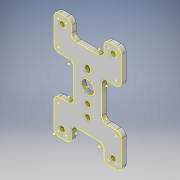
# Autodesk Inventor part: TapaInferior
Saved by Autodesk Inventor 2019 (Build 230136000, 136)
## iProperties
Created: 2019-03-04
Part Number: TapaInferior
Material: Generic
Document SubType Name: Modeling
Designer: Kenny
Density: 1 g/cm^3
Appearance: Default
Author: Kenny
Autodesk Inventor part; units mm, degrees
ref_plane "YZ Plane" through (0, 0, 0) normal (1, 0, 0) x (0, 1, 0)
ref_plane "XZ Plane" through (0, 0, 0) normal (0, 1, 0) x (-1, 0, 0)
ref_plane "XY Plane" through (0, 0, 0) normal (0, 0, 1) x (1, 0, 0)
sketch "Sketch1" plane through (0, 0, 0) normal (0, 0, 1) x (1, 0, 0)
  line L0 (41, 0) -> (41, 65.3) construction
  line L1 (0, 65.3) -> (0, 0) construction
  line L2 (41, 0) -> (41, 21)
  line L3 (0, 21) -> (0, 0)
  line L4 (41, 65.3) -> (41, 44.3)
  line L5 (0, 44.3) -> (0, 65.3)
  line L6 (29, 44.3) -> (29, 21)
  line L7 (12, 21) -> (12, 44.3)
  line L8 (41, 44.3) -> (29, 44.3)
  line L9 (12, 44.3) -> (0, 44.3)
  line L10 (41, 21) -> (29, 21)
  line L11 (12, 21) -> (0, 21)
  line L12 (30.5, 65.3) -> (30.5, 55.3)
  line L13 (30.5, 55.3) -> (10.5, 55.3)
  line L14 (10.5, 55.3) -> (10.5, 65.3)
  line L15 (41, 65.3) -> (30.5, 65.3) construction
  line L16 (10.5, 65.3) -> (0, 65.3) construction
  line L17 (0, 65.3) -> (10.5, 65.3)
  line L18 (30.5, 65.3) -> (41, 65.3)
  line L19 (10.5, 0) -> (10.5, 10)
  line L20 (10.5, 10) -> (30.5, 10)
  line L21 (30.5, 10) -> (30.5, 0)
  line L22 (0, 0) -> (10.5, 0) construction
  line L23 (30.5, 0) -> (41, 0) construction
  line L24 (0, 0) -> (10.5, 0)
  line L25 (30.5, 0) -> (41, 0)
  circle A0 centre (20.5, 35) radius 4
  point P0 (5, 60.3)
  point P1 (36, 60.3)
  point P2 (5, 5)
  point P3 (36, 5)
  point P4 (20.5, 44)
  point P5 (20.5, 26)
  point P6 (20.5, 19)
  point P7 (20.5, 45)
  dimension "d0" = 41
  dimension "d1" = 65.3
  dimension "d2" = 21
  dimension "d3" = 21
  dimension "d4" = 12
  dimension "d5" = 9
  dimension "d6" = 9
  dimension "d7" = 7
  dimension "d8" = 1
  dimension "d9" = 5
  dimension "d11" = 5
  dimension "d12" = 41
  dimension "d13" = 41
  dimension "d14" = 12
  dimension "d15" = 10.5
  dimension "d16" = 10.5
  dimension "d17" = 8
  dimension "d18" = 20.5
  dimension "d19" = 5
  dimension "d20" = 5
  constraints: 52 end point, 18 parallel, 10 vertical alignment, 6 horizontal, 6 perpendicular, 2 horizontal alignment, 1 centre point, 1 coincident
  measures "d0" distance of L1.start L0.end
  measures "d1" distance of L0.end L0.start
  measures "d2" distance of L2.end L2.start
  measures "d3" distance of L4.start L4.end
  measures "d4" distance between parallel lines of L0 L6
  measures "d5" distance of point (20.5, 35) point (20.5, 44)
  measures "d6" distance of point (20.5, 26) point (20.5, 35)
  measures "d7" distance of point (20.5, 19) point (20.5, 26)
  measures "d8" distance of point (20.5, 44) point (20.5, 45)
  measures "d9" distance from line of L1 point (5, 60.3)
  measures "d11" distance from line of L0 point (36, 60.3)
  measures "d12" distance between parallel lines of L1 L2
  measures "d13" distance between parallel lines of L1 L4
  measures "d14" distance between parallel lines of L3 L7
  measures "d15" distance between parallel lines of L5 L14
  measures "d16" distance between parallel lines of L0 L12
  measures "d17" diameter of A0
  measures "d18" distance from line of L3 point (20.5, 19)
  measures "d19" distance from line of L16 point (5, 60.3)
  measures "d20" distance from line of L22 point (5, 5)
extrude "Extrusion1" add sketch "Sketch1" along normal blind 3
sketch "Sketch2" plane through (0, 0, 0) normal (0, 0, 1) x (1, 0, 0)
  line L0 (41, 0) -> (41, 65.3) construction
  line L1 (0, 65.3) -> (0, 0) construction
  line L2 (41, 0) -> (41, 21)
  line L3 (0, 21) -> (0, 0)
  line L4 (41, 65.3) -> (41, 44.3)
  line L5 (0, 44.3) -> (0, 65.3)
  line L6 (29, 44.3) -> (29, 21)
  line L7 (12, 21) -> (12, 44.3)
  line L8 (41, 44.3) -> (29, 44.3)
  line L9 (12, 44.3) -> (0, 44.3)
  line L10 (41, 21) -> (29, 21)
  line L11 (12, 21) -> (0, 21)
  line L12 (30.5, 65.3) -> (30.5, 55.3)
  line L13 (30.5, 55.3) -> (10.5, 55.3)
  line L14 (10.5, 55.3) -> (10.5, 65.3)
  line L15 (41, 65.3) -> (30.5, 65.3) construction
  line L16 (10.5, 65.3) -> (0, 65.3) construction
  line L17 (0, 65.3) -> (10.5, 65.3)
  line L18 (30.5, 65.3) -> (41, 65.3)
  line L19 (10.5, 0) -> (10.5, 10)
  line L20 (10.5, 10) -> (30.5, 10)
  line L21 (30.5, 10) -> (30.5, 0)
  line L22 (0, 0) -> (10.5, 0) construction
  line L23 (30.5, 0) -> (41, 0) construction
  line L24 (0, 0) -> (10.5, 0)
  line L25 (30.5, 0) -> (41, 0)
  circle A0 centre (20.5, 35) radius 4
  point P0 (5, 60.3)
  point P1 (36, 60.3)
  point P2 (5, 5)
  point P3 (36, 5)
  point P4 (20.5, 44)
  point P5 (20.5, 26)
  point P6 (20.5, 19)
  point P7 (20.5, 45)
  dimension "d21" = 41
  dimension "d22" = 65.3
  dimension "d23" = 21
  dimension "d24" = 21
  dimension "d25" = 12
  dimension "d28" = 7
  dimension "d29" = 1
  dimension "d30" = 5
  dimension "d31" = 5
  dimension "d32" = 41
  dimension "d33" = 41
  dimension "d34" = 12
  dimension "d35" = 10.5
  dimension "d36" = 10.5
  dimension "d37" = 8
  dimension "d38" = 20.5
  dimension "d39" = 5
  dimension "d40" = 5
  constraints: 52 end point, 18 parallel, 8 vertical alignment, 6 horizontal, 6 perpendicular, 2 horizontal alignment, 1 centre point
  measures "d21" distance of L1.start L0.end
  measures "d22" distance of L0.end L0.start
  measures "d23" distance of L2.end L2.start
  measures "d24" distance of L4.start L4.end
  measures "d25" distance between parallel lines of L0 L6
  measures "d28" distance of point (20.5, 19) point (20.5, 26)
  measures "d29" distance of point (20.5, 44) point (20.5, 45)
  measures "d30" distance from line of L1 point (5, 60.3)
  measures "d31" distance from line of L0 point (36, 60.3)
  measures "d32" distance between parallel lines of L1 L2
  measures "d33" distance between parallel lines of L1 L4
  measures "d34" distance between parallel lines of L3 L7
  measures "d35" distance between parallel lines of L5 L14
  measures "d36" distance between parallel lines of L0 L12
  measures "d37" diameter of A0
  measures "d38" distance from line of L3 point (20.5, 19)
  measures "d39" distance from line of L16 point (5, 60.3)
  measures "d40" distance from line of L22 point (5, 5)
hole "Hole1" at (5, 60.3, 0) at (36, 60.3, 0) at (5, 5, 0) at (36, 5, 0) at (20.5, 44, 0) at (20.5, 26, 0) at (20.5, 19, 0) at (20.5, 45, 0) direction (0, 0, 1) diameter 3.3 end through all
fillet "Fillet1" radius 3 20 edges at (10.5, 65.3, 1.5) (0, 65.3, 1.5) (0, 44.3, 1.5) (12, 44.3, 1.5) (12, 21, 1.5) (0, 21, 1.5) (0, 0, 1.5) (10.5, 0, 1.5) (10.5, 10, 1.5) (30.5, 10, 1.5) (30.5, 0, 1.5) (41, 0, 1.5) (41, 21, 1.5) (29, 21, 1.5) (29, 44.3, 1.5) (41, 44.3, 1.5) (41, 65.3, 1.5) (30.5, 65.3, 1.5) (30.5, 55.3, 1.5) (10.5, 55.3, 1.5)
sketch "Sketch3" plane through (0, 0, 3) normal (0, 0, 1) x (1, 0, 0)
  line L0 (22.15, 45) -> (22.15, 44)
  arc A0 (18.9276, 44.5) -> (22.0724, 44.5) centre (20.5, 44) ccw projected
  arc A1 (22.0724, 44.5) -> (18.9276, 44.5) centre (20.5, 45) ccw projected
  line L1 (18.85, 45) -> (18.85, 44)
  point P0 (0, 0)
  constraints: 4 end point, 4 point on circle, 4 tangent, 1 vertical
extrude "Extrusion2" cut sketch "Sketch3" against normal blind 3 contours L0 A0 A1 | A1 A0 L1
sketch "Sketch4" plane through (0, 0, 3) normal (0, 0, 1) x (1, 0, 0)
  circle A0 centre (20.5, 35) radius 4 projected
  circle A1 centre (20.5, 26) radius 1.65 projected
  circle A2 centre (36, 5) radius 1.65 projected
  circle A3 centre (36, 60.3) radius 1.65 projected
  circle A4 centre (5, 60.3) radius 1.65 projected
  circle A5 centre (5, 5) radius 1.65 projected
  line L0 (22.15, 45) -> (22.15, 44) projected
  arc A6 (18.85, 44) -> (22.15, 44) centre (20.5, 44) ccw projected
  line L1 (18.85, 44) -> (18.85, 45) projected
  arc A7 (22.15, 45) -> (18.85, 45) centre (20.5, 45) ccw projected
  circle A8 centre (20.5, 19) radius 1.65 projected
  arc A9 (33.5, 65.3) -> (30.5, 62.3) centre (33.5, 62.3) ccw projected
  line L2 (30.5, 62.3) -> (30.5, 58.3) projected
  arc A10 (27.5, 55.3) -> (30.5, 58.3) centre (27.5, 58.3) ccw projected
  line L3 (27.5, 55.3) -> (13.5, 55.3) projected
  arc A11 (10.5, 58.3) -> (13.5, 55.3) centre (13.5, 58.3) ccw projected
  line L4 (10.5, 58.3) -> (10.5, 62.3) projected
  arc A12 (10.5, 62.3) -> (7.5, 65.3) centre (7.5, 62.3) ccw projected
  line L5 (7.5, 65.3) -> (3, 65.3) projected
  arc A13 (3, 65.3) -> (0, 62.3) centre (3, 62.3) ccw projected
  line L6 (0, 62.3) -> (0, 47.3) projected
  arc A14 (0, 47.3) -> (3, 44.3) centre (3, 47.3) ccw projected
  line L7 (3, 44.3) -> (9, 44.3) projected
  arc A15 (12, 41.3) -> (9, 44.3) centre (9, 41.3) ccw projected
  line L8 (12, 41.3) -> (12, 24) projected
  arc A16 (9, 21) -> (12, 24) centre (9, 24) ccw projected
  line L9 (9, 21) -> (3, 21) projected
  arc A17 (3, 21) -> (0, 18) centre (3, 18) ccw projected
  line L10 (0, 18) -> (0, 3) projected
  arc A18 (0, 3) -> (3, 0) centre (3, 3) ccw projected
  line L11 (3, 0) -> (7.5, 0) projected
  arc A19 (7.5, 0) -> (10.5, 3) centre (7.5, 3) ccw projected
  line L12 (10.5, 3) -> (10.5, 7) projected
  arc A20 (13.5, 10) -> (10.5, 7) centre (13.5, 7) ccw projected
  line L13 (13.5, 10) -> (27.5, 10) projected
  arc A21 (30.5, 7) -> (27.5, 10) centre (27.5, 7) ccw projected
  line L14 (30.5, 7) -> (30.5, 3) projected
  arc A22 (30.5, 3) -> (33.5, 0) centre (33.5, 3) ccw projected
  line L15 (33.5, 0) -> (38, 0) projected
  arc A23 (38, 0) -> (41, 3) centre (38, 3) ccw projected
  line L16 (41, 3) -> (41, 18) projected
  arc A24 (41, 18) -> (38, 21) centre (38, 18) ccw projected
  line L17 (38, 21) -> (32, 21) projected
  arc A25 (29, 24) -> (32, 21) centre (32, 24) ccw projected
  line L18 (29, 24) -> (29, 41.3) projected
  arc A26 (32, 44.3) -> (29, 41.3) centre (32, 41.3) ccw projected
  line L19 (32, 44.3) -> (38, 44.3) projected
  arc A27 (38, 44.3) -> (41, 47.3) centre (38, 47.3) ccw projected
  line L20 (41, 47.3) -> (41, 62.3) projected
  arc A28 (41, 62.3) -> (38, 65.3) centre (38, 62.3) ccw projected
  line L21 (38, 65.3) -> (33.5, 65.3) projected
  point P0 (0, 0)
body "Solid1"
